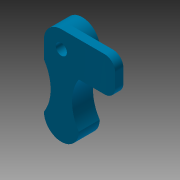
# Autodesk Inventor part: glass clip
Saved by Autodesk Inventor 2015 (Build 190159000, 159)
## iProperties
Created: 2015-07-09
Part Number: glass clip
Material: ABS Plastic
Document SubType Name: Modeling
Designer: hp
Density: 1.06 g/cm^3
Appearance: Sky Blue Medium
Author: hp
Autodesk Inventor part; units mm, degrees
ref_plane "YZ Plane" through (0, 0, 0) normal (1, 0, 0) x (0, 1, 0)
ref_plane "XZ Plane" through (0, 0, 0) normal (0, 1, 0) x (-1, 0, 0)
ref_plane "XY Plane" through (0, 0, 0) normal (0, 0, 1) x (1, 0, 0)
sketch "Sketch1" plane through (0, 0, 0) normal (0, 1, 0) x (-1, 0, 0)
  line L0 (0, 5) -> (-12.44, 5)
  line L1 (-15.44, 2) -> (-15.44, -2)
  line L2 (-12.44, -5) -> (5, -5)
  line L3 (5, -5) -> (5, 0)
  arc A0 (-12.44, 5) -> (-15.44, 2) centre (-12.44, 2) ccw
  arc A1 (-15.44, -2) -> (-12.44, -5) centre (-12.44, -2) ccw
  arc A2 (5, 0) -> (0, 5) centre (0, 0) ccw
  point P0 (-15.44, -5)
  point P1 (-15.44, 5)
  dimension "d0" = 20.44
  dimension "d1" = 10
  dimension "d2" = 3
  dimension "d3" = 5
  constraints: 8 end point, 6 point on circle, 6 tangent, 4 point on line, 3 centre point, 2 parallel, 1 coincident, 1 equal radius, 1 horizontal, 1 perpendicular
  measures "d0" distance of L2.end point (-15.44, -5)
  measures "d1" distance of point (-15.44, -5) point (-15.44, 5)
  measures "d2" radius of A0
  measures "d3" radius of A2
extrude "Extrusion1" add sketch "Sketch1" along normal blind 2.35
sketch "Sketch3" plane through (0, 0, 0) normal (0, -1, 0) x (1, 0, 0)
  arc A0 (5, 0) -> (-5, 0) centre (0, 0) ccw
  arc A1 (-5, -18) -> (5, -18) centre (0, -18) ccw
  line L0 (-5, 0) -> (-5, -5)
  line L1 (5, 0) -> (5, -5)
  arc A2 (-5, -18) -> (-5, -5) centre (-15, -11.5) ccw
  arc A3 (5, -5) -> (5, -18) centre (15, -11.5) ccw
  dimension "d6" = 5
  dimension "d7" = 18
  dimension "d8" = 5
  dimension "d9" = 5
  dimension "d11" = 15
  dimension "d12" = 15
  constraints: 8 point on circle, 4 centre point, 4 end point, 3 horizontal alignment, 1 coincident, 1 vertical, 1 vertical alignment
  measures "d6" radius of A1
  measures "d7" distance of point (0, 0) A1.centre
  measures "d8" distance of L0.start L0.end
  measures "d9" distance of L1.start L1.end
  measures "d11" horizontal distance of point (0, 0) A3.centre
  measures "d12" horizontal distance of point (0, 0) A2.centre
extrude "Extrusion2" add sketch "Sketch3" against normal blind 6
sketch "Sketch4" plane through (0, 6, 0) normal (0, 1, 0) x (1, 0, 0)
  circle A0 centre (0, 0) radius 1.6
  dimension "d16" = 3.2
  constraints: 1 centre point, 1 coincident
  measures "d16" diameter of A0
extrude "Extrusion3" cut sketch "Sketch4" against normal up to next
body "Solid1"
